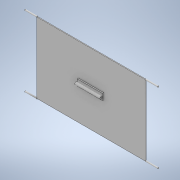
# Autodesk Inventor part: Bandeja
Saved by Autodesk Inventor 2021 (Build 250183000, 183)
## iProperties
Created: 2021-04-19
Part Number: Bandeja
Material: Genérico
Document SubType Name: Modeling
Designer: carlo
Density: 1 g/cm^3
Appearance: Valor por defecto
Author: carlo
Autodesk Inventor part; units mm, degrees
ref_plane "YZ Plane" through (0, 0, 0) normal (1, 0, 0) x (0, 1, 0)
ref_plane "XZ Plane" through (0, 0, 0) normal (0, 1, 0) x (-1, 0, 0)
ref_plane "XY Plane" through (0, 0, 0) normal (0, 0, 1) x (1, 0, 0)
sketch "Boceto1" plane through (0, 0, 0) normal (0, 0, 1) x (1, 0, 0)
  line L0 (-215, 140) -> (215, 140)
  line L1 (215, 140) -> (215, -140)
  line L2 (215, -140) -> (-215, -140)
  line L3 (-215, -140) -> (-215, 140)
  line L4 (-215, 140) -> (215, -140) construction
  line L5 (215, 140) -> (-215, -140) construction
  point P0 (0, 0)
  dimension "d0" = 430
  dimension "d1" = 280
  constraints: 12 end point, 2 midpoint, 2 parallel, 1 horizontal, 1 perpendicular
  measures "d0" distance of L1.end L2.end
  measures "d1" distance of L0.end L1.end
extrude "Extrusión1" add sketch "Boceto1" along normal blind 3
sketch "Boceto2" plane through (0, 0, 3) normal (0, 0, 1) x (1, 0, 0)
  line L0 (-50, -12.5) -> (50, -12.5)
  line L1 (50, -12.5) -> (50, 12.5)
  line L2 (50, 12.5) -> (-50, 12.5)
  line L3 (-50, 12.5) -> (-50, -12.5)
  line L4 (-50, -12.5) -> (50, 12.5) construction
  line L5 (50, -12.5) -> (-50, 12.5) construction
  point P0 (0, 0)
  dimension "d4" = 100
  dimension "d5" = 25
  constraints: 12 end point, 2 midpoint, 2 parallel, 1 horizontal, 1 perpendicular
  measures "d4" distance of L2.end L1.end
  measures "d5" distance of L1.end L0.end
extrude "Extrusión2" add sketch "Boceto2" along normal blind 5
sketch "Boceto3" plane through (50, -12.5, 3) normal (1, 0, 0) x (0, 0, -1)
  line L0 (-5, 0) -> (-5, 12.5)
  circle A0 centre (-10, 12.5) radius 5
  circle A1 centre (-10, 12.5) radius 2.5
  point P0 (3, 12.5)
  dimension "d10" = 5
  constraints: 2 end point, 1 centre point, 1 coincident, 1 horizontal alignment, 2 other
  measures "d10" diameter of A1
extrude "Extrusión3" add sketch "Boceto3" against normal blind 100
sketch "Boceto11" plane through (215, -140, 0) normal (1, 0, 0) x (0, 0, -1)
  line L0 (0, 280) -> (-3, 280) projected
  circle A0 centre (-1.5, 280) radius 2.5
  line L1 (0, 0) -> (-3, 0) projected
  circle A1 centre (-1.5, 0) radius 2.5
  point P0 (0, 140)
  dimension "d31" = 5
  dimension "d32" = 5
  constraints: 2 centre point, 2 midpoint
  measures "d31" diameter of A0
  measures "d32" diameter of A1
extrude "Extrusión8" add sketch "Boceto11" along normal blind 50
sketch "Boceto12" plane through (-215, -140, 0) normal (-1, 0, 0) x (0, 0, 1)
  line L0 (0, 0) -> (3, 0) projected
  circle A0 centre (1.5, 0) radius 2.5
  line L1 (0, 280) -> (3, 280) projected
  circle A1 centre (1.5, 280) radius 2.5
  point P0 (0, 140)
  dimension "d35" = 5
  dimension "d36" = 5
  constraints: 2 centre point, 2 midpoint
  measures "d35" diameter of A0
  measures "d36" diameter of A1
extrude "Extrusión9" add sketch "Boceto12" along normal blind 47.58
